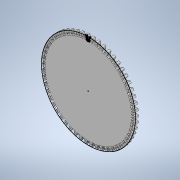
# Autodesk Inventor part: GearUberBig54T
Saved by Autodesk Inventor 2022 (Build 260153070, 153G)
## iProperties
Created: 2021-11-03
Part Number: GearUberBig54T
Material: Generic
Document SubType Name: Modeling
Designer: a laptop
Density: 1 g/cm^3
Appearance: Default
Author: a laptop
Autodesk Inventor part; units mm, degrees
ref_plane "YZ Plane" through (0, 0, 0) normal (1, 0, 0) x (0, 1, 0)
ref_plane "XZ Plane" through (0, 0, 0) normal (0, 1, 0) x (-1, 0, 0)
ref_plane "XY Plane" through (0, 0, 0) normal (0, 0, 1) x (1, 0, 0)
sketch "Sketch1" plane through (0, 0, 0) normal (0, 0, 1) x (1, 0, 0)
  spline S0 degree 3 poles (-1.6175, 41.9688) (-1.4995, 41.6273) (-1.3225, 41.115) (-1.152, 40.4116) (-1.1097, 40.0527) (-1.0886, 39.8733) knots 0 0 0 0 0.10835 0.162535 0.21669 0.21669 0.21669 0.21669
  spline S1 degree 3 poles (-1.0886, 39.8733) (-1.0835, 39.7056) (-1.0759, 39.454) (-1.0178, 39.1224) (-0.9351, 38.9276) (-0.8377, 38.7893) (-0.7383, 38.7109) (-0.6286, 38.6466) (-0.3776, 38.6032) (0, 38.6425) (0.3776, 38.6032) (0.6286, 38.6466) (0.7383, 38.7109) (0.8377, 38.7893) (0.9351, 38.9276) (1.0178, 39.1224) (1.0759, 39.454) (1.0835, 39.7056) (1.0886, 39.8733) knots 0 0 0 0 0.050275 0.075433 0.100524 0.113112 0.125681 0.138249 0.150797 0.201123 0.251449 0.263997 0.276565 0.289134 0.301722 0.326813 0.351971 0.402246 0.402246 0.402246 0.402246
  spline S2 degree 3 poles (1.0886, 39.8733) (1.1097, 40.0527) (1.152, 40.4116) (1.3225, 41.115) (1.4995, 41.6273) (1.6175, 41.9688) knots 0 0 0 0 0.054155 0.10834 0.21669 0.21669 0.21669 0.21669
  circle A0 centre (0, 0) radius 38.625 construction
  circle A1 centre (0, 0) radius 39.8847 construction
  circle A2 centre (0, 0) radius 40.5 construction
  circle A3 centre (0, 0) radius 42
  point P0 (-1.2854, 40.9375)
  point P1 (-1.1627, 40.4097)
  point P2 (-1.0574, 39.3715)
  point P3 (-1.0084, 39.1247)
  point P4 (-0.9082, 38.8947)
  point P5 (-0.8333, 38.7935)
  point P6 (-0.7366, 38.7133)
  point P7 (-0.6259, 38.6537)
  point P8 (-0.5033, 38.6272)
  point P9 (0, 38.625)
  point P10 (0.5033, 38.6272)
  point P11 (0.6259, 38.6537)
  point P12 (0.7366, 38.7133)
  point P13 (0.8333, 38.7935)
  point P14 (0.9082, 38.8947)
  point P15 (1.0084, 39.1247)
  point P16 (1.0574, 39.3715)
  point P17 (1.1627, 40.4097)
  point P18 (1.2854, 40.9375)
  constraints: 4 centre point, 2 point on circle, 53 other
extrude "Extrusion1" add sketch "Sketch1" against normal blind 3
extrude "Extrusion2" cut sketch "Sketch1" against normal blind 10 contours A3 S2 S1 S0 picked at (0.3629, 40.5828)
pattern_circular "Circular Pattern1" count 54 over 360 about axis through (0, 0, 0) along (0, 0, -1) of "Extrusion2"
equation "\"d0\" = FaceWidth"
equation "\"Module\" = 1.5"
equation "\"PressureAngle\" = 10deg"
equation "\"UnitProfileClearance\" = 0.25"
equation "\"UnitRoundRadius\" = 0.3025"
equation "\"HeadDiameter\" = 84"
equation "\"RootDiameter\" = 77.25"
equation "\"BaseDiameter\" = 79.76943"
equation "\"PitchDiameter\" = 81"
equation "\"FaceWidth\" = 3"
equation "\"HelixAngle\" = 0"
equation "\"UnitCorrection\" = 0"
equation "\"UnitAddendumModification\" = 0"
equation "\"CircularPitch\" = 4.712389"
equation "\"UnitBacklashShift\" = 0"
equation "\"TotalToolShift\" = 0"
equation "\"IsInternal\" = 0"
body "Solid1"
